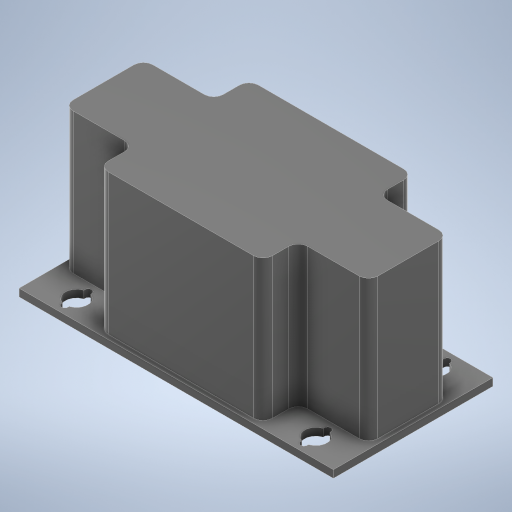
# Autodesk Inventor part: SUSTAINA-POWER-DISTRIBUTION-BOARD
Saved by Autodesk Inventor 2024.2 (Build 282272000, 272)
## iProperties
Created: 2024-01-24
Part Number: SUSTAINA-POWER-DISTRIBUTION-BOARD
Material: Acetal Resin, Black
Document SubType Name: Modeling
Designer: Masato Kubotera
Appearance: Smooth - Black
Surface Area: 123.153 cm^2
Volume: 52.2328 cm^3
Author: Masato Kubotera
Autodesk Inventor part; units mm, degrees
ref_plane "YZ Plane" through (0, 0, 0) normal (1, 0, 0) x (0, 1, 0)
ref_plane "XZ Plane" through (0, 0, 0) normal (0, 1, 0) x (-1, 0, 0)
ref_plane "XY Plane" through (0, 0, 0) normal (0, 0, 1) x (1, 0, 0)
sketch "Sketch1" plane through (0, 0, 0) normal (0, 0, 1) x (1, 0, 0)
  line L0 (17, 33.5) -> (-17, 33.5)
  line L1 (-17, 33.5) -> (-17, -33.5)
  line L2 (-17, -33.5) -> (17, -33.5)
  line L3 (17, -33.5) -> (17, 33.5)
  line L4 (17, 33.5) -> (-17, -33.5) construction
  line L5 (-17, 33.5) -> (17, -33.5) construction
  line L6 (-12.75, 25.5) -> (12.75, 25.5) construction
  line L7 (12.75, 25.5) -> (12.75, -25.5) construction
  line L8 (12.75, -25.5) -> (-12.75, -25.5) construction
  line L9 (-12.75, -25.5) -> (-12.75, 25.5) construction
  line L10 (-12.75, 25.5) -> (12.75, -25.5) construction
  line L11 (12.75, 25.5) -> (-12.75, -25.5) construction
  line L12 (17, 0) -> (-17, 0) construction
  line L13 (0, 33.5) -> (0, -33.5) construction
  circle A0 centre (12.75, 25.5) radius 2.4
  circle A1 centre (-12.75, 25.5) radius 2.4
  circle A2 centre (12.75, -25.5) radius 2.4
  circle A3 centre (-12.75, -25.5) radius 2.4
  line L14 (12.75, 32.5) -> (12.75, 18.5) construction
  line L15 (16, 17.5) -> (-16, 17.5)
  line L16 (-16, 17.5) -> (-16, -17.5)
  line L17 (-16, -17.5) -> (16, -17.5)
  line L18 (16, -17.5) -> (16, 17.5)
  line L19 (16, 17.5) -> (-16, -17.5) construction
  line L20 (-16, 17.5) -> (16, -17.5) construction
  line L21 (8.5, 17.5) -> (8.5, 32.5)
  line L22 (8.5, 32.5) -> (-8.5, 32.5)
  line L23 (-8.5, 32.5) -> (-8.5, 17.5)
  line L24 (8.5, -17.5) -> (8.5, -32.5)
  line L25 (8.5, -32.5) -> (-8.5, -32.5)
  line L26 (-8.5, -32.5) -> (-8.5, -17.5)
  arc A4 (10.4605, 26.2199) -> (10.4605, 24.7801) centre (10.25, 25.5) ccw
  arc A5 (15.0395, 24.7801) -> (15.0395, 26.2199) centre (15.25, 25.5) ccw
  arc A6 (10.4605, -24.7801) -> (10.4605, -26.2199) centre (10.25, -25.5) ccw
  arc A7 (15.0395, -26.2199) -> (15.0395, -24.7801) centre (15.25, -25.5) ccw
  arc A8 (-10.4605, 24.7801) -> (-10.4605, 26.2199) centre (-10.25, 25.5) ccw
  arc A9 (-15.0395, 26.2199) -> (-15.0395, 24.7801) centre (-15.25, 25.5) ccw
  arc A10 (-10.4605, -26.2199) -> (-10.4605, -24.7801) centre (-10.25, -25.5) ccw
  arc A11 (-15.0395, -24.7801) -> (-15.0395, -26.2199) centre (-15.25, -25.5) ccw
  point P0 (0, 0)
  point P1 (8.5, -17.5)
  point P2 (-8.5, -17.5)
  point P3 (16, 25.5)
  point P4 (9.5, 25.5)
  point P5 (15.0395, 26.2199)
  point P6 (15.0395, 24.7801)
  point P7 (15.0395, -24.7801)
  point P8 (15.0395, -26.2199)
  point P9 (10.4605, -26.2199)
  point P10 (10.4605, -24.7801)
  point P11 (-15.0395, -26.2199)
  point P12 (-15.0395, -24.7801)
  point P13 (-10.4605, -24.7801)
  point P14 (-10.4605, -26.2199)
  point P15 (-15.0395, 24.7801)
  point P16 (-15.0395, 26.2199)
  point P17 (-10.4605, 26.2199)
  point P18 (-10.4605, 24.7801)
  dimension "d0" = 34
  dimension "d1" = 67
  dimension "d19" = 4.8
  dimension "d33" = 51
  dimension "d34" = 25.5
  dimension "d38" = 1
  dimension "d43" = 1
  dimension "d44" = 1
  dimension "d46" = 6.5
  dimension "d47" = 1.5
  dimension "d48" = 1
  dimension "d50" = 16
  constraints: 54 end point, 28 symmetric about line, 20 point on circle, 12 centre point, 11 midpoint, 6 coincident, 6 parallel, 4 horizontal, 3 perpendicular, 3 point on line, 3 vertical, 13 other
  measures "d0" distance of L2.end L1.end
  measures "d1" distance of L1.end L0.end
  measures "d19" diameter of A0
  measures "d33" distance of L8.end L6.start
  measures "d34" distance of L7.end L8.end
  measures "d38" distance between parallel lines of L3 L18
  measures "d43" distance from line of L0 L14.start
  measures "d44" distance between parallel lines of L0 L22
  measures "d46" distance of point (16, 25.5) point (9.5, 25.5)
  measures "d47" diameter of A4
  measures "d48" distance from line of L3 point (16, 25.5)
  measures "d50" diameter of L0 L6
extrude "Extrusion1" add sketch "Sketch1" along normal blind 1.6 contours L3 L2 L1 L0 | L18 L17 L16 L15 | L15 L23 L22 L21 | L24 L25 L26 L17
extrude "Extrusion2" add sketch "Sketch1" along normal blind 31.6 contours L18 L17 L16 L15 | L15 L23 L22 L21 | L24 L25 L26 L17
fillet "Fillet1" radius 2 12 edges at (16, -17.5, 16.6) (16, 17.5, 16.6) (-16, -17.5, 16.6) (-16, 17.5, 16.6) (8.5, 17.5, 16.6) (8.5, -17.5, 16.6) (8.5, -32.5, 16.6) (-8.5, -32.5, 16.6) (-8.5, -17.5, 16.6) (-8.5, 17.5, 16.6) (-8.5, 32.5, 16.6) (8.5, 32.5, 16.6)
body "Solid1"
